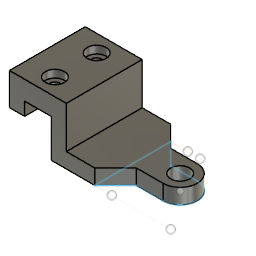
MaRS_Q5_b (Autodesk Fusion 360 design; units mm, degrees)
part number: 2026-05-26-12-02-48-327
Autodesk Fusion 360 part; units mm, degrees
sketch "Sketch1" plane through (0, 0, 0) normal (0, 1, 0) x (1, 0, 0)
  line L0 (0, -150) -> (0, -65)
  line L1 (0, -65) -> (40, -65)
  line L2 (40, -65) -> (40, -100)
  line L3 (0, 0) -> (225, 0)
  line L4 (225, -40) -> (225, 0)
  line L5 (40, -100) -> (110, -100)
  line L6 (0, -150) -> (150, -150)
  line L7 (110, -100) -> (110, 0)
  line L8 (150, -150) -> (150, -40)
  line L9 (150, -40) -> (225, -40)
  dimension "d7" = 150
  dimension "d9" = 85
  dimension "d11" = 35
  dimension "d14" = 225
  dimension "d15" = 70
  dimension "d16" = 150
  dimension "d17" = 110
  constraint perpendicular L0 L1
  constraint perpendicular L1 L2
  constraint coincident L3.start origin
  constraint horizontal L3
  constraint perpendicular L3 L4
  constraint perpendicular L2 L5
  constraint perpendicular L0 L6
  constraint coincident L3 L7.end
  constraint perpendicular L3 L7
  constraint perpendicular L6 L8
  constraint perpendicular L4 L9
  measures "d7" distance of L3.start L0.start
  measures "d9" distance of L0.start L0.end
  measures "d11" distance of L1.end L2.end
  measures "d14" distance of L3.start L3.end
  measures "d15" distance of L2.end L5.end
  measures "d16" distance of L0.start L6.end
  measures "d17" distance of L6.end L8.end
extrude "Extrude1" add sketch "Sketch1" along normal blind 200
sketch "Sketch2" plane through (0, 0, 0) normal (0, 0, 1) x (1, 0, 0)
  line L0 (224.8321, 0) -> (425, 0) construction
  line L1 (225, 200) -> (270, 200) construction
  line L2 (224.8321, 0) -> (269.8321, 0) construction
  line L3 (350, 145) -> (280, 145)
  line L4 (350.0871, 55.0001) -> (279.6959, 54.8638)
  line L5 (225, 200) -> (280, 145)
  line L6 (225, 200) -> (302.7817, 200) construction
  line L7 (224.8321, 0) -> (256.6519, 31.8198)
  line L8 (256.6519, 31.8198) -> (279.6959, 54.8638)
  arc A0 (350.0871, 55.0001) -> (350, 145) centre (350, 100) ccw
  line L9 (225, 200) -> (224.8321, 0)
  dimension "d24" = 90
  dimension "d29" = 45
  dimension "d30" = 45
  constraint horizontal L0
  constraint horizontal L1
  constraint horizontal L2
  constraint tangent L3 A0
  constraint tangent L4 A0
  constraint horizontal L6
  constraint parallel L7 L8
  measures "d24" diameter of A0
  measures "d29" angle of L5 L6
  measures "d30" distance of L0.start L7.end
extrude "Extrude2" add sketch "Sketch2" along normal blind 40
sketch "Sketch3" plane through (0, 0, 40) normal (0, 0, 1) x (-1, 0, 0)
  line L0 (-150, 0) -> (-225, 0)
  line L1 (-225, 0) -> (-225, -0.1679)
  line L2 (-225, -0.1679) -> (-279.6959, -54.8638)
  line L3 (-279.6959, -54.8638) -> (-350.0871, -55.0001)
  arc A0 (-350.0871, -55.0001) -> (-350, -145) centre (-350, -100) ccw
  line L4 (-350, -145) -> (-280, -145)
  line L5 (-280, -145) -> (-225, -200)
  line L6 (-225, -200) -> (-150, -200)
  line L7 (-150, -200) -> (-150, 0)
  circle A1 centre (-350, -100) radius 25
  constraint concentric A0 A1
extrude "Extrude3" cut sketch "Sketch3" against normal blind 40 contours A1
sketch "Sketch4" plane through (0, 0, 150) normal (0, 0, 1) x (-1, 0, 0)
  line L0 (0, 0) -> (-150, 0)
  line L1 (-150, 0) -> (-150, -200)
  line L2 (-150, -200) -> (0, -200)
  line L3 (0, -200) -> (0, 0)
  circle A0 centre (-75, -155) radius 25
  circle A1 centre (-75, -45) radius 25
extrude "Extrude4" cut sketch "Sketch4" against normal blind 20 contours A0 | A1
sketch "Sketch5" plane through (0, 0, 150) normal (0, 0, 1) x (-1, 0, 0)
  circle A0 centre (-75, -155) radius 25
  circle A1 centre (-75, -45) radius 25
  line L0 (0, 0) -> (-150, 0)
  line L1 (-150, 0) -> (-150, -200)
  line L2 (-150, -200) -> (0, -200)
  line L3 (0, -200) -> (0, 0)
  circle A2 centre (-75, -155) radius 12.5
  circle A3 centre (-75, -45) radius 12.5
  dimension "d43" = 25
  dimension "d44" = 25
  constraint concentric A0 A2
  constraint concentric A1 A3
  measures "d43" diameter of A2
  measures "d44" diameter of A3
extrude "Extrude5" cut sketch "Sketch5" against normal blind 80 contours A2 | A3
extrude "Extrude6" add sketch "Sketch2" along normal blind 40
sketch "Sketch6" plane through (0, 0, 40) normal (0, 0, 1) x (-1, 0, 0)
  line L0 (-150, 0) -> (-225, 0)
  line L1 (-225, 0) -> (-225, -0.1679)
  line L2 (-225, -0.1679) -> (-279.6959, -54.8638)
  line L3 (-279.6959, -54.8638) -> (-350.0871, -55.0001)
  arc A0 (-350.0871, -55.0001) -> (-350, -145) centre (-350, -100) ccw
  line L4 (-350, -145) -> (-280, -145)
  line L5 (-280, -145) -> (-225, -200)
  line L6 (-225, -200) -> (-150, -200)
  line L7 (-150, -200) -> (-150, 0)
  circle A1 centre (-350, -100) radius 25
  dimension "d49" = 50
  constraint concentric A0 A1
  measures "d49" diameter of A1
extrude "Extrude7" cut sketch "Sketch6" against normal blind 60 contours A1
